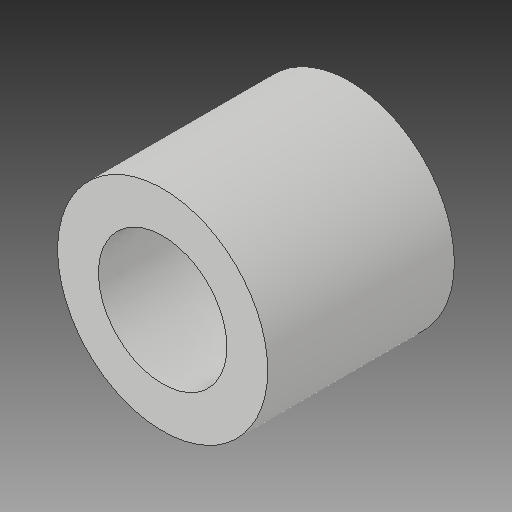
# Autodesk Inventor part: 8mm Rumba Spacer
Saved by Autodesk Inventor 2018 (Build 220112000, 112)
## iProperties
Created: 2016-07-28
Part Number: 8mm Rumba Spacer
Material: Generic
Document SubType Name: Modeling
Designer: User
Density: 1 g/cm^3
Appearance: Default
Author: User
Autodesk Inventor part; units mm, degrees
ref_plane "YZ Plane" through (0, 0, 0) normal (1, 0, 0) x (0, 1, 0)
ref_plane "XZ Plane" through (0, 0, 0) normal (0, 1, 0) x (-1, 0, 0)
ref_plane "XY Plane" through (0, 0, 0) normal (0, 0, 1) x (1, 0, 0)
sketch "Sketch1" plane through (0, 0, 0) normal (0, 0, 1) x (1, 0, 0)
  arc A0 (-43.2697, -2.2187) -> (-43.4396, -1.8087) centre (-44.9118, -2.6587) ccw projected
  circle A1 centre (-44.9118, -2.6587) radius 2.75
  circle A2 centre (-44.9118, -2.6587) radius 4.5
  point P0 (0, 0)
  dimension "d0" = 5.5
  dimension "d1" = 9
  constraints: 2 centre point, 2 coincident
  measures "d0" diameter of A1
  measures "d1" diameter of A2
extrude "Extrusion1" add sketch "Sketch1" along normal blind 8
body "Solid1"
